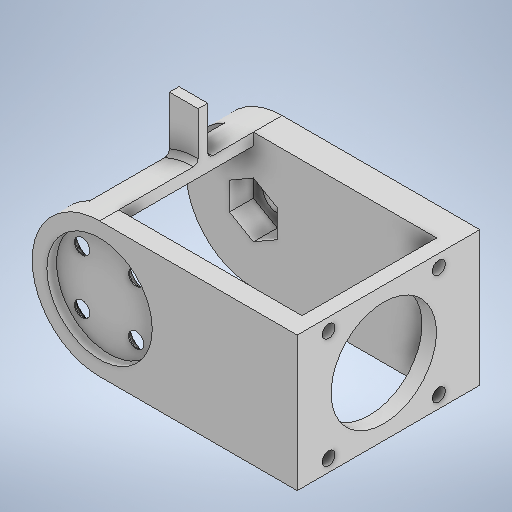
# Autodesk Inventor part: j6 motor mount v2
Saved by Autodesk Inventor 2025 (Build 290162000, 162)
## iProperties
Created: 2025-08-05
Part Number: j6 motor mount v2
Material: 一般
Document SubType Name: Modeling
Designer: gavin
Density: 1 g/cm^3
Appearance: 預設
Author: gavin
## iProperties of the stored document j6 motor mount v2_3D 列印.ipt
Created: 2025-08-05
Part Number: j6 motor mount v2_3D 列印
Material: 一般
Document SubType Name: Modeling
Designer: gavin
Density: 1 g/cm^3
Appearance: 預設
Author: gavin
Autodesk Inventor part; units mm, degrees
ref_plane "YZ Plane" through (0, 0, 0) normal (1, 0, 0) x (0, 1, 0)
ref_plane "XZ Plane" through (0, 0, 0) normal (0, 1, 0) x (-1, 0, 0)
sketch "草圖1" plane through (0, 0, 0) normal (1, 0, 0) x (0, 1, 0)
  line L0 (-14.075, 14.075) -> (14.075, 14.075)
  line L1 (14.075, 14.075) -> (14.075, -14.075)
  line L2 (14.075, -14.075) -> (-14.075, -14.075)
  line L3 (-14.075, -14.075) -> (-14.075, 14.075)
  line L4 (-14.075, 14.075) -> (14.075, -14.075) construction
  line L5 (14.075, 14.075) -> (-14.075, -14.075) construction
  line L6 (14.075, 14.075) -> (-14.075, 14.075)
  line L7 (-14.075, 14.075) -> (-14.075, 18.075)
  line L8 (-14.075, 18.075) -> (14.075, 18.075)
  line L9 (14.075, 18.075) -> (14.075, 14.075)
  circle A0 centre (0, 0) radius 11
  line L10 (-11.5, 11.5) -> (11.5, 11.5) construction
  line L11 (11.5, 11.5) -> (11.5, -11.5) construction
  line L12 (11.5, -11.5) -> (-11.5, -11.5) construction
  line L13 (-11.5, -11.5) -> (-11.5, 11.5) construction
  line L14 (-11.5, 11.5) -> (11.5, -11.5) construction
  line L15 (11.5, 11.5) -> (-11.5, -11.5) construction
  circle A1 centre (11.5, 11.5) radius 1.35
  circle A2 centre (-11.5, 11.5) radius 1.35
  circle A3 centre (-11.5, -11.5) radius 1.35
  circle A4 centre (11.5, -11.5) radius 1.35
  line L16 (14.075, -14.075) -> (-14.075, -14.075)
  line L17 (-14.075, -14.075) -> (-14.075, -20.075)
  line L18 (-14.075, -20.075) -> (14.075, -20.075)
  line L19 (14.075, -20.075) -> (14.075, -14.075)
  dimension "d0" = 28.15
  dimension "d1" = 28.15
  dimension "d2" = 4
  dimension "d3" = 22
  dimension "d4" = 23
  dimension "d5" = 23
  dimension "d6" = 2.7
  dimension "d9" = 360
  dimension "d11" = 6
  constraints: 40 end point, 8 parallel, 5 centre point, 4 horizontal, 4 midpoint, 4 perpendicular, 2 coincident, 9 other
  measures "d0" distance of L1.end L2.end
  measures "d1" distance of L0.end L1.end
  measures "d2" distance of L6.end L7.end
  measures "d3" diameter of A0
  measures "d4" distance of L11.end L12.end
  measures "d5" distance of L10.end L11.end
  measures "d6" diameter of A1
  measures "d11" distance of L17.end L16.end
extrude "擠出1" add sketch "草圖1" along normal blind 3
sketch "草圖2" plane through (0, 0, 0) normal (-1, 0, 0) x (0, 0, 1)
  line L0 (18.075, 14.075) -> (18.075, -14.075) projected
  line L1 (-20.075, 14.075) -> (18.075, 14.075) projected
  line L2 (-20.075, -14.075) -> (-20.075, 14.075) projected
  line L3 (18.075, -14.075) -> (-20.075, -14.075) projected
  circle A0 centre (0, 0) radius 11 projected
  circle A1 centre (11.5, 11.5) radius 1.35 projected
  circle A2 centre (11.5, -11.5) radius 1.35 projected
  circle A3 centre (-11.5, -11.5) radius 1.35 projected
  circle A4 centre (-11.5, 11.5) radius 1.35 projected
  line L4 (-14.075, 14.075) -> (-14.075, -14.075)
  line L5 (14.075, 14.075) -> (14.075, -14.075)
  dimension "d14" = 6
  dimension "d15" = 4
  constraints: 4 end point, 4 point on line, 2 vertical
  measures "d14" distance between parallel lines of L2 L4
  measures "d15" distance between parallel lines of L0 L5
extrude "擠出2" add sketch "草圖2" along normal blind 52.375 contours L0 L3 L5 L1 | L4 L3 L2 L1
sketch "草圖3" plane through (3, -14.075, 18.075) normal (0, 0, 1) x (1, 0, 0)
  line L0 (-55.375, 0) -> (0, 0) projected
  line L1 (0, 28.15) -> (0, 0) projected
  line L2 (0, 28.15) -> (-55.375, 28.15) projected
  line L3 (-55.375, 0) -> (-55.375, 28.15) projected
  circle A0 centre (-41.3, 14.075) radius 11
  line L4 (-55.375, 0) -> (-55.375, 28.15) projected
  circle A1 centre (-41.3, 14.075) radius 8 construction
  line L5 (-41.3, 14.075) -> (-33.5218, 21.8532) construction
  line L6 (-41.3, 14.075) -> (-30.3, 14.075) construction
  circle A2 centre (-35.6431, 19.7319) radius 1.6
  circle A3 centre (-46.9569, 19.7319) radius 1.6
  circle A4 centre (-46.9569, 8.4181) radius 1.6
  circle A5 centre (-35.6431, 8.4181) radius 1.6
  point P0 (-3, 14.075)
  dimension "d18" = 22
  dimension "d19" = 16
  dimension "d65" = 10
  dimension "d20" = 45
  dimension "d21" = 3.2
  dimension "d24" = 360
  dimension "d30" = 14.075
  dimension "d31" = 14.075
  constraints: 4 centre point, 4 end point, 1 coincident, 1 equal length, 1 horizontal, 1 horizontal alignment, 1 point on line, 15 other
  measures "d20" angle of L6 L5
  measures "d21" diameter of A2
  measures "d30" distance from line of L2 point (-41.3, 14.075)
  measures "d31" distance from line of L3 point (-41.3, 14.075)
extrude "擠出3" cut sketch "草圖3" against normal up to surface (4 mm away) contours A2 | A3 | A4 | A5
extrude "擠出4" cut sketch "草圖3" against normal blind 2 contours A0
fillet "圓角1" radius 14.075 4 edges at (-52.375, 14.075, 16.075) (-52.375, 14.075, -17.075) (-52.375, -14.075, 16.075) (-52.375, -14.075, -17.075)
sketch "草圖4" plane through (0, -14.075, -14.075) normal (0, 0, 1) x (1, 0, 0)
  circle A0 centre (-38.3, 14.075) radius 11 projected
  line L0 (-38.3, 8.3015) -> (-43.3, 11.1882)
  line L1 (-43.3, 11.1882) -> (-43.3, 16.9618)
  line L2 (-43.3, 16.9618) -> (-38.3, 19.8485)
  line L3 (-38.3, 19.8485) -> (-33.3, 16.9618)
  line L4 (-33.3, 16.9618) -> (-33.3, 11.1882)
  line L5 (-33.3, 11.1882) -> (-38.3, 8.3015)
  point P0 (0, 14.075)
  dimension "d33" = 10
  constraints: 12 end point, 1 coincident, 13 other
  measures "d33" distance between parallel lines of L4 L1
extrude "擠出5" cut sketch "草圖4" against normal blind 5 contours L0 L1 L2 L3 L4 L5
sketch "草圖5" plane through (0, -14.075, -19.075) normal (0, 0, 1) x (1, 0, 0)
  circle A0 centre (-38.3, 14.075) radius 11 projected
  circle A1 centre (-38.3, 14.075) radius 3.1
  point P0 (0, 14.075)
  dimension "d36" = 6.2
  constraints: 1 centre point, 1 coincident
  measures "d36" diameter of A1
extrude "擠出6" cut sketch "草圖5" against normal up to surface (1 mm away) contours A1
sketch "草圖7" plane through (3, 0, 0) normal (1, 0, 0) x (0, 0, -1)
  line L0 (-18.075, 14.075) -> (-18.075, -14.075) projected
  line L1 (-18.075, -14.075) -> (20.075, -14.075) projected
  line L2 (20.075, -14.075) -> (20.075, 14.075) projected
  line L3 (20.075, 14.075) -> (-18.075, 14.075) projected
  circle A0 centre (0, 0) radius 11 projected
  circle A1 centre (-11.5, 11.5) radius 1.35 projected
  circle A2 centre (-11.5, -11.5) radius 1.35 projected
  circle A3 centre (11.5, -11.5) radius 1.35 projected
  circle A4 centre (11.5, 11.5) radius 1.35 projected
  line L4 (-2.75, 14.075) -> (-2.75, 10.6507)
  line L5 (2.75, 14.075) -> (2.75, 10.6507)
  dimension "d44" = 5.5
  dimension "d45" = 2.75
  constraints: 4 end point, 2 point on circle, 2 point on line, 2 vertical
  measures "d44" distance between parallel lines of L5 L4
  measures "d45" distance from line of point (0, 0) L5
chamfer "倒角1" distance 1.8 angle 45 4 edges at (-45.5569, -5.6569, 14.075) (-45.5569, 5.6569, 14.075) (-34.2431, -5.6569, 14.075) (-34.2431, 5.6569, 14.075)
sketch "草圖11" plane through (3, -14.075, 18.075) normal (0, 0, 1) x (1, 0, 0)
  line L0 (-37.3248, 33.6873) -> (-37.3375, 43.4872) projected
  line L1 (-37.3248, 33.6873) -> (-31.2248, 33.6951) projected
  line L2 (-31.2375, 43.4951) -> (-31.2248, 33.6951) projected
  line L3 (-37.3375, 43.4872) -> (-31.2375, 43.4951) projected
  arc A0 (-41.3, 28.15) -> (-41.3, 0) centre (-41.3, 14.075) ccw projected
  line L4 (-41.3, 0) -> (0, 0) projected
  line L5 (0, 28.15) -> (0, 0) projected
  line L6 (0, 28.15) -> (-41.3, 28.15) projected
  circle A1 centre (-41.3, 14.075) radius 11 projected
  line L7 (-31.2003, 28.15) -> (-31.2003, 25.65)
  line L8 (-31.2003, 25.65) -> (-47.301, 25.65)
  line L9 (-47.301, 25.65) -> (-47.301, 26.8066)
  line L10 (-41.3, 28.15) -> (-41.3, 25.65)
  point P0 (-3, 14.075)
  dimension "d64" = 2.5
  constraints: 8 end point, 3 perpendicular, 2 point on line, 1 point on circle, 1 vertical
  measures "d64" distance between parallel lines of L8 L6
extrude "擠出12" add sketch "草圖11" against normal up to surface (38.15 mm away) contours L10 L8 L9 A0
ref_plane "工作平面4" through (3, -14.075, -3.53) normal (0, 0, 1) x (1, 0, 0)
sketch "草圖15" plane through (3, -14.075, -3.53) normal (0, 0, 1) x (1, 0, 0)
  line L0 (0, 28.15) -> (-41.3, 28.15) projected
  arc A0 (-41.3, 28.15) -> (-41.3, 0) centre (-41.3, 14.075) ccw projected
  line L1 (-47.3274, 33.6866) -> (-47.3385, 41.6466) construction
  line L2 (-47.3274, 33.6866) -> (-41.2274, 33.6951) construction
  line L3 (-41.2385, 41.6551) -> (-41.2274, 33.6951) construction
  line L4 (-47.3385, 41.6466) -> (-41.2385, 41.6551) construction
  line L5 (-41.3, 38.15) -> (-47.301, 38.15)
  line L6 (-41.3, 38.15) -> (-41.3, 28.15)
  line L7 (-47.301, 38.15) -> (-47.301, 26.8066)
  point P0 (-3, 14.075)
  point P1 (-47.301, 26.8066)
  dimension "d78" = 10
  constraints: 6 end point, 2 vertical, 2 vertical alignment, 1 horizontal, 1 point on circle, 1 point on line
  measures "d78" distance of L5.start L6.end
extrude "擠出16" add sketch "草圖15" along normal mid plane 2
fillet "圓角5" radius 1 2 edges at (-41.3748, 13.735, -4.53) (-41.3748, 13.735, -2.53)
equation "\"d31\" = d30"
equation "\"d26\" = d19"
equation "\"d45\" = 0.5 * d44"
